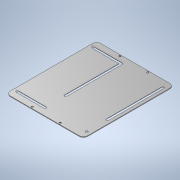
# Autodesk Inventor part: PlateLateral
Saved by Autodesk Inventor 2022 (Build 260153000, 153)
## iProperties
Created: 2022-12-14
Part Number: PlateLateral
Material: Aluminum, Anodized Silver
Document SubType Name: Modeling
Designer: braxt
Density: 2.7 g/cm^3
Appearance: Anodized - Light Gray
Description: Aluminum Plate 6061: T651, 24 in Overall Lg, 24 in Overall Wd, 0.25 in Thick, Mill, +/-0.012 in
Stock Number: 2HGR5
Author: braxt
Autodesk Inventor part; units mm, degrees
ref_plane "YZ Plane" through (0, 0, 0) normal (1, 0, 0) x (0, 1, 0)
ref_plane "XZ Plane" through (0, 0, 0) normal (0, 1, 0) x (-1, 0, 0)
ref_plane "XY Plane" through (0, 0, 0) normal (0, 0, 1) x (1, 0, 0)
sketch "Sketch1" plane through (0, 0, 0) normal (0, 1, 0) x (-1, 0, 0)
  line L0 (-613.8, 55) -> (-513.8, 55)
  line L1 (-387.5, 55) -> (-613.8, 55)
  line L2 (-513.8, 55) -> (-473.8, 55)
  line L3 (-469.3, 380.5) -> (-343, 380.5)
  line L4 (-343, 390.5) -> (-469.3, 390.5)
  line L5 (-474.3, 385.5) -> (-474.3, 385.5)
  circle A0 centre (-658.3, 385.5) radius 5
  arc A1 (-474.3, 385.5) -> (-469.3, 380.5) centre (-469.3, 385.5) ccw
  arc A2 (-469.3, 390.5) -> (-474.3, 385.5) centre (-469.3, 385.5) ccw
  line L6 (-513.8, 395) -> (-513.8, 395.5)
  line L7 (-513.8, 55) -> (-469.3, 55)
  line L8 (-474.3, 65) -> (-474.3, 65)
  line L9 (-474.3, 178.5) -> (-474.3, 178.5)
  line L10 (-474.3, 292) -> (-474.3, 292)
  line L11 (-653.3, 45) -> (-653.3, 272)
  line L12 (-663.3, 45) -> (-663.3, 272)
  line L13 (-613.8, 395.5) -> (-513.8, 395.5)
  line L14 (-513.8, 395.5) -> (-513.8, 168.5)
  line L15 (-513.8, 168.5) -> (-613.8, 168.5)
  line L16 (-513.8, 168.5) -> (-387.5, 168.5)
  line L17 (-613.8, 168.5) -> (-613.8, 395.5)
  line L18 (-513.8, 395.5) -> (-513.8, 29.6)
  line L19 (-613.8, 29.6) -> (-613.8, 168.5)
  line L20 (-387.5, 29.6) -> (-387.5, 395.5)
  line L21 (-387.5, 395.5) -> (-513.8, 395.5)
  line L22 (-387.5, 29.6) -> (-613.8, 29.6)
  line L23 (-513.8, 282) -> (-613.8, 282)
  line L24 (-663.3, 45) -> (-663.3, 39.6)
  line L25 (-653.3, 39.6) -> (-653.3, 45)
  arc A3 (-663.3, 39.6) -> (-653.3, 39.6) centre (-658.3, 39.6) ccw
  line L26 (-663.3, 272) -> (-663.3, 292)
  line L27 (-653.3, 292) -> (-653.3, 272)
  arc A4 (-653.3, 292) -> (-663.3, 292) centre (-658.3, 292) ccw
  line L28 (-464.3, 292) -> (-464.3, 183.5)
  line L29 (-474.3, 178.5) -> (-474.3, 292)
  arc A5 (-464.3, 292) -> (-474.3, 292) centre (-469.3, 292) ccw
  line L30 (-474.3, 183.5) -> (-474.3, 65)
  line L31 (-464.3, 70) -> (-464.3, 292)
  arc A6 (-343, 34.6) -> (-343, 44.6) centre (-343, 39.6) ccw
  line L32 (-343, 34.6) -> (-369.3, 34.6)
  line L33 (-364.3, 44.6) -> (-343, 44.6)
  line L34 (-369.3, 34.6) -> (-364.3, 34.6)
  line L35 (-663.3, 183.5) -> (-676.3, 183.5)
  line L36 (-676.3, 6.6) -> (-676.3, 418.5)
  line L37 (-324.4347, 22.1004) -> (-324.4347, 40.1004)
  line L38 (-324.4127, 6.6) -> (-324.9989, 418.5)
  arc A7 (-343, 380.5) -> (-343, 390.5) centre (-343, 385.5) ccw
  line L39 (-613.8, 55) -> (-613.8, 395.5)
  line L40 (-474.3, 65) -> (-474.3, 39.6)
  line L41 (-469.3, 34.6) -> (-369.3, 34.6)
  line L42 (-464.3, 70) -> (-464.3, 44.6)
  line L43 (-464.3, 44.6) -> (-364.3, 44.6)
  arc A8 (-474.3, 39.6) -> (-469.3, 34.6) centre (-469.3, 39.6) ccw
  line L44 (-437.15, 411.5) -> (-564.15, 411.5)
  line L45 (-437.15, 13.6) -> (-564.15, 13.6)
  line L46 (-324.4127, 6.6) -> (-676.3, 6.6)
  line L47 (-676.3, 418.5) -> (-324.9989, 418.5)
  point P0 (-469.3, 178.5)
  point P1 (-469.3, 292)
  point P2 (-474.3, 385.5)
  dimension "d9" = 10
  dimension "d75" = 126.3
  dimension "d76" = 226.3
  dimension "d78" = 10
  dimension "d79" = 10
  dimension "d82" = 10
  dimension "d92" = 10
  dimension "d98" = 13
  dimension "d205" = 365.9
  dimension "d206" = 227
  dimension "d207" = 340.5
  dimension "d208" = 5
  dimension "d238" = 127
  dimension "d240" = 127
  constraints: 96 end point, 16 point on circle, 9 centre point, 8 point on line, 7 parallel, 6 horizontal, 6 tangent, 4 perpendicular, 4 vertical, 2 collinear, 1 midpoint
  measures "d9" diameter of A0
  measures "d75" distance of L18.end L20.start
  measures "d76" distance of L20.start L19.start
  measures "d78" diameter of A3
  measures "d79" diameter of A4
  measures "d82" diameter of A5
  measures "d92" diameter of A6
  measures "d98" distance of L35.start L35.end
  measures "d205" distance of L20.start L20.end
  measures "d206" distance of L15.end L13.start
  measures "d207" distance of L0.start L13.start
  measures "d208" radius of A8
  measures "d238" distance of L44.start L44.end
  measures "d240" distance of L45.start L45.end
extrude "Extrusion1" add sketch "Sketch1" along normal blind 3.175 contours L19 L15 L18 L0 | L0 L18 L22 L19 | L18 L16 L30 L40 L1 | L1 L40 A8 L41 L20 L22 L18 | L17 L23 L14 L15 | L14 L6 L21 L20 L4 A2 A1 L3 L16 L31 L28 A5 L29 L30 | L17 L13 L6 L14 L23 | L16 L20 L1 L42 L31 | L1 L20 L43 L42 | L36 L47 L38 L46
sketch "Sketch2" plane through (0, 0, 0) normal (0, -1, 0) x (1, 0, 0)
  line L0 (474.3, 178.5) -> (474.3, 178.5)
  line L1 (513.8, 168.5) -> (413.8, 168.5)
  line L2 (413.8, 395.5) -> (413.8, 55)
  line L3 (513.8, 395.5) -> (513.8, 29.6)
  line L4 (387.5, 29.6) -> (387.5, 395.5)
  line L5 (474.3, 65) -> (474.3, 65)
  line L6 (474.3, 385.5) -> (474.3, 385.5)
  line L7 (513.8, 395) -> (513.8, 395.5)
  line L8 (613.8, 29.6) -> (613.8, 168.5)
  line L9 (613.8, 55) -> (513.8, 55)
  line L10 (513.8, 55) -> (473.8, 55)
  line L11 (513.8, 55) -> (469.3, 55)
  line L12 (413.8, 55) -> (613.8, 55)
  line L13 (613.8, 168.5) -> (613.8, 395.5)
  line L14 (513.8, 395.5) -> (513.8, 168.5)
  line L15 (513.8, 168.5) -> (613.8, 168.5)
  line L16 (474.3, 292) -> (474.3, 292)
  line L17 (387.5, 29.6) -> (613.8, 29.6)
  line L18 (513.8, 282) -> (613.8, 282)
  line L19 (387.5, 395.5) -> (513.8, 395.5)
  line L20 (613.8, 395.5) -> (513.8, 395.5)
  line L21 (475.3, 378.5) -> (337, 378.5)
  line L22 (337, 392.5) -> (475.3, 392.5)
  circle A0 centre (658.3, 385.5) radius 7.75
  line L23 (665.3, 272) -> (665.3, 298)
  line L24 (651.3, 298) -> (651.3, 272)
  line L25 (651.3, 272) -> (651.3, 45)
  line L26 (651.3, 45) -> (651.3, 33.6)
  line L27 (665.3, 33.6) -> (665.3, 45)
  line L28 (665.3, 45) -> (665.3, 272)
  line L29 (369.3, 32.6) -> (337, 32.6)
  line L30 (337, 46.6) -> (355.3, 46.6)
  line L31 (462.3, 79) -> (462.3, 164.5)
  line L32 (462.3, 192.5) -> (462.3, 298)
  line L33 (476.3, 65) -> (476.3, 183.5)
  line L34 (476.3, 178.5) -> (476.3, 298)
  arc A1 (476.3, 298) -> (462.3, 298) centre (469.3, 298) ccw
  arc A2 (337, 46.6) -> (337, 32.6) centre (337, 39.6) ccw
  arc A3 (651.3, 33.6) -> (665.3, 33.6) centre (658.3, 33.6) ccw
  arc A4 (665.3, 298) -> (651.3, 298) centre (658.3, 298) ccw
  arc A5 (475.3, 378.5) -> (475.3, 392.5) centre (475.3, 385.5) ccw
  arc A6 (337, 392.5) -> (337, 378.5) centre (337, 385.5) ccw
  line L35 (476.3, 65) -> (476.3, 39.6)
  line L36 (469.3, 32.6) -> (369.3, 32.6)
  line L37 (343, 34.6) -> (469.3, 34.6) projected
  line L38 (462.3, 79) -> (462.3, 53.6)
  line L39 (464.3, 44.6) -> (343, 44.6) projected
  line L40 (455.3, 46.6) -> (355.3, 46.6)
  arc A7 (469.3, 32.6) -> (476.3, 39.6) centre (469.3, 39.6) ccw
  arc A8 (455.3, 46.6) -> (462.3, 53.6) centre (455.3, 53.6) ccw
  line L41 (462.3, 164.5) -> (462.3, 192.5)
  line L42 (464.3, 292) -> (464.3, 44.6) projected
  line L43 (676.3, 11.6) -> (324.4127, 11.6) projected
  line L44 (324.4127, 6.6) -> (324.9989, 418.5) projected
  line L45 (325, 413.5) -> (676.3, 413.5) projected
  line L46 (676.3, 418.5) -> (676.3, 6.6) projected
  point P0 (650, 0)
  point P1 (0, 41.6)
  point P2 (0, 378.5)
  point P3 (413.8, 282)
  point P4 (469.3, 178.5)
  point P5 (676.3, 450)
  point P6 (676.3, 0)
  point P7 (513.8, 55)
  point P8 (513.8, 29.6)
  point P9 (362.3, 46.6)
  point P10 (462.3, 72)
  point P11 (462.3, 171.5)
  point P12 (462.3, 185.5)
  point P13 (376.3, 58)
  point P14 (325, 424)
  point P15 (324.9989, 418.5)
  dimension "d178" = 15.5
  dimension "d186" = 14
  dimension "d190" = 14
  dimension "d192" = 14
  dimension "d194" = 14
  dimension "d198" = 14
  dimension "d202" = 14
  dimension "d209" = 7
  constraints: 80 end point, 16 point on circle, 9 centre point, 9 point on line, 4 tangent, 2 parallel, 2 perpendicular, 1 equal radius, 1 vertical, 1 other
  measures "d178" diameter of A0
  measures "d186" diameter of A1
  measures "d190" diameter of A2
  measures "d192" diameter of A3
  measures "d194" diameter of A4
  measures "d198" diameter of A5
  measures "d202" diameter of A6
  measures "d209" radius of A7
extrude "Extrusion2" cut sketch "Sketch2" against normal blind 2 contours L33 L35 L10 L11 L12 L42 L1 | L1 L41 L32 A1 L34 L33 | L42 L12 L38 L31 L41 L1 | L35 A7 L36 L4 L39 L42 L12 L11 L10 | L42 L39 L4 L40 A8 L38 L12 | L36 L29 A2 L30 L40 L4 | L21 L4 L22 L2 | L2 L22 A5 L21 | L21 A6 L22 L4 | A0 | L28 L27 A3 L26 L25 L24 A4 L23
fillet "Fillet1" radius 20 4 edges at (324.4127, 1.5875, 6.6) (676.3, 1.5875, 6.6) (676.3, 1.5875, 418.5) (324.9989, 1.5875, 418.5)
hole "Hole2" at (437.15, 0, 13.6) at (564.15, 0, 13.6) at (437.15, 0, 411.5) at (564.15, 0, 411.5) direction (0, 1, 0) diameter 8 end through all counterbore diameter 12 counterbore depth 2
body "Solid1"
